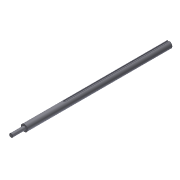
# Autodesk Inventor part: ShooterAxle
Saved by Autodesk Inventor 2012 (Build 160160000, 160)
## iProperties
Created: 2012-02-21
Part Number: ShooterAxle
Material: Steel
Document SubType Name: Modeling
Designer: JesseK
Mass: 277.503 g
Surface Area: 125.045 cm^2
Volume: 35.3507 cm^3
Density: 7.85 g/cm^3
Author: JesseK
Autodesk Inventor part; units mm, degrees
ref_plane "YZ Plane" through (0, 0, 0) normal (1, 0, 0) x (0, 1, 0)
ref_plane "XZ Plane" through (0, 0, 0) normal (0, 1, 0) x (-1, 0, 0)
ref_plane "XY Plane" through (0, 0, 0) normal (0, 0, 1) x (1, 0, 0)
sketch "Sketch1" plane through (0, 0, 0) normal (0, 0, 1) x (1, 0, 0)
  circle A0 centre (0, 0) radius 6.35
  dimension "d0" = 12.7
  constraints: 1 centre point, 1 coincident
  measures "d0" diameter of A0
extrude "Extrusion1" add sketch "Sketch1" along normal blind 304.8
sketch "Sketch2" plane through (0, 0, 304.8) normal (0, 0, 1) x (1, 0, 0)
  circle A0 centre (0, 0) radius 6.35 projected
  circle A1 centre (0, 0) radius 3.429
  circle A2 centre (0, 0) radius 6.35
  dimension "d3" = 6.858
  constraints: 2 centre point, 2 coincident, 1 concentric
  measures "d3" diameter of A1
extrude "Extrusion2" cut sketch "Sketch2" against normal blind 25.4
sketch "Sketch3" plane through (0, 0, 0) normal (0, 0, -1) x (-1, 0, 0)
  circle A0 centre (0, 0) radius 6.35 projected
  arc A1 (1.5875, 6.1484) -> (-1.5875, 6.1484) centre (0, 0) ccw
  line L0 (-1.5875, 6.1484) -> (-1.5875, 4.7625)
  line L1 (-1.5875, 4.7625) -> (1.5875, 4.7625)
  line L2 (1.5875, 4.7625) -> (1.5875, 6.1484)
  line L3 (0, 6.35) -> (1.0636, 6.35) construction
  dimension "d6" = 3.175
  dimension "d7" = 1.5875
  constraints: 8 end point, 3 horizontal, 3 point on circle, 2 vertical, 1 centre point, 1 coincident, 1 parallel, 1 tangent, 2 other
  measures "d6" distance of L0.end L1.end
  measures "d7" distance between parallel lines of L1 L3
extrude "Extrusion3" cut sketch "Sketch3" against normal blind 203.2 contours L2 L1 L0 A0 picked at (0.1781, 5.2842)
body "Solid1"
